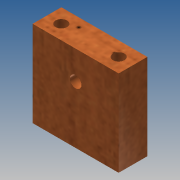
# Autodesk Inventor part: hubjig_tab
Saved by Autodesk Inventor 2014 SP1 (Build 180222100, 222)
## iProperties
Created: 2014-08-29
Part Number: hubjig_tab
Material: Wood (Cherry)
Document SubType Name: Modeling
Designer: Dave
Mass: 11.6143 g
Surface Area: 48.387 cm^2
Volume: 18.4354 cm^3
Density: 0.63 g/cm^3
Appearance: Cherry - Natural Low Gloss
Author: Dave
Autodesk Inventor part; units mm, degrees
ref_plane "YZ Plane" through (0, 0, 0) normal (1, 0, 0) x (0, 1, 0)
ref_plane "XZ Plane" through (0, 0, 0) normal (0, 1, 0) x (-1, 0, 0)
ref_plane "XY Plane" through (0, 0, 0) normal (0, 0, 1) x (1, 0, 0)
sketch "Sketch1" plane through (0, 0, 0) normal (0, 1, 0) x (-1, 0, 0)
  line L0 (0, 0) -> (38.1, 0)
  line L1 (38.1, 0) -> (38.1, 12.7)
  line L2 (38.1, 12.7) -> (0, 12.7)
  line L3 (0, 12.7) -> (0, 0)
  dimension "d0" = 38.1
  dimension "d1" = 12.7
  constraints: 8 end point, 2 parallel, 1 horizontal, 1 perpendicular
  measures "d0" distance of L0.start L0.end
  measures "d1" distance of L2.end L0.start
extrude "Extrusion1" add sketch "Sketch1" along normal blind 38.1
sketch "Sketch2" plane through (0, 38.1, 0) normal (0, 1, 0) x (1, 0, 0)
  line L0 (0, 0) -> (-38.1, 0) projected
  line L1 (-38.1, -12.7) -> (0, -12.7) projected
  line L2 (-19.05, 0) -> (-19.05, -12.7) construction
  circle A0 centre (-31.75, -6.35) radius 3.7798
  circle A1 centre (-6.35, -6.35) radius 3.7798
  dimension "d4" = 12.7
  constraints: 2 centre point, 2 end point, 2 midpoint, 1 symmetric about line, 1 other
  measures "d4" distance from line of L2 A0.centre
hole "Hole1" at (-31.75, 38.1, 6.35) at (-6.35, 38.1, 6.35) direction (0, -1, 0) diameter 5.1054 end through all clearance for "Flat Head Machine Screw (82)" size "#10" standard "Ansi Unified Screw Threads"
sketch "Sketch3" plane through (-38.1, 0, 12.7) normal (0, 0, 1) x (1, 0, 0)
  line L0 (0, 38.1) -> (38.1, 38.1) projected
  circle A0 centre (19.05, 25.4) radius 3.652
  dimension "d12" = 12.7
  constraints: 1 centre point
  measures "d12" distance from line of A0.centre L0
hole "Hole2" at (-19.05, 25.4, 12.7) direction (0, 0, -1) diameter 5.1054 end through all clearance for "Flat Head Machine Screw (82)" size "#10" standard "Ansi Unified Screw Threads"
body "Solid1"
